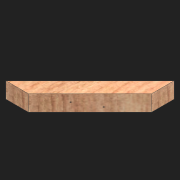
# Autodesk Inventor part: C002
Saved by Autodesk Inventor 2017 SP1 (Build 210196100, 196)
## iProperties
Created: 2017-06-13
Part Number: C002
Material: Wood (Birch)
Document SubType Name: Modeling
Designer: zallen
Density: 0.55 g/cm^3
Appearance: Birch - Natural Polished
Mass: 30.515 g
Surface Area: 153.189 cm^2
Volume: 11.3018 cm^3
Author: zallen
Autodesk Inventor part; units mm, degrees
ref_plane "YZ Plane" through (0, 0, 0) normal (1, 0, 0) x (0, 1, 0)
ref_plane "XZ Plane" through (0, 0, 0) normal (0, 1, 0) x (-1, 0, 0)
ref_plane "XY Plane" through (0, 0, 0) normal (0, 0, 1) x (1, 0, 0)
sketch "Sketch1" plane through (0, 0, 0) normal (0, 0, 1) x (1, 0, 0)
  line L0 (0, 0) -> (100, 0) construction
  line L1 (100, 0) -> (100, 100) construction
  line L2 (100, 100) -> (0, 100) construction
  line L3 (0, 100) -> (0, 0) construction
  line L4 (0, 0) -> (100, 100)
  line L5 (0, 0) -> (26.9408, 0)
  line L6 (100, 100) -> (100, 73.0592)
  line L7 (26.9408, 0) -> (100, 73.0592)
  dimension "d1" = 100
  dimension "d2" = 100
  dimension "d35" = 19.05
  constraints: 16 end point, 2 parallel, 2 point on line, 1 horizontal, 1 perpendicular
  measures "d1" distance of L2.end L1.end
  measures "d2" distance of L1.end L0.end
  measures "d35" distance between parallel lines of L7 L4
extrude "Extrusion1" add sketch "Sketch1" along normal blind 19.05
body "Solid1"
